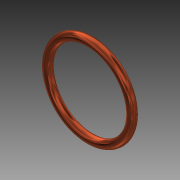
# Autodesk Inventor part: 21xx_WireLoop_2,1mm_Inner
Saved by Autodesk Inventor 2021 (Build 250183000, 183)
## iProperties
Created: 2022-06-20
Part Number: 21xx_WireLoop_2,1mm_Inner
Material: Copper, Cast
Document SubType Name: Modeling
Designer: Eli
Density: 8.94 g/cm^3
Appearance: Copper - Satin
Author: Eli
Autodesk Inventor part; units mm, degrees
ref_plane "YZ Plane" through (0, 0, 0) normal (1, 0, 0) x (0, 1, 0)
ref_plane "XZ Plane" through (0, 0, 0) normal (0, 1, 0) x (-1, 0, 0)
ref_plane "XY Plane" through (0, 0, 0) normal (0, 0, 1) x (1, 0, 0)
sketch "Sketch1" plane through (0, 0, 0) normal (1, 0, 0) x (0, 1, 0)
  circle A0 centre (10.75, 0) radius 1.05
  line L0 (0, -1.47) -> (0, 1.47) projected
  point P0 (0, 0)
  dimension "d0" = 2.1
  dimension "d1" = 10.75
  constraints: 1 centre point, 1 horizontal alignment
  measures "d0" diameter of A0
  measures "d1" distance of point (0, 0) A0.centre
revolve "Revolution1" add sketch "Sketch1" angle 360 about axis through (0, 0, -10) along (0, 0, 1)
pattern_linear "Rectangular Pattern1" count 6 spacing 2.1 along (0, 0, 1) of "Revolution1"
body "Solid1"
